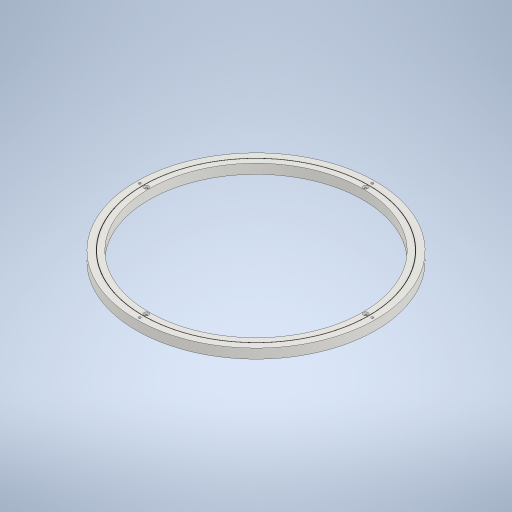
# Autodesk Inventor part: bearing_table
Saved by Autodesk Inventor 2023 (Build 270158000, 158)
## iProperties
Created: 2023-03-04
Part Number: bearing_table
Material: Generic
Document SubType Name: Modeling
Designer: caleb
Density: 1 g/cm^3
Appearance: Default
Author: caleb
Autodesk Inventor part; units mm, degrees
ref_plane "YZ Plane" through (0, 0, 0) normal (1, 0, 0) x (0, 1, 0)
ref_plane "XZ Plane" through (0, 0, 0) normal (0, 1, 0) x (-1, 0, 0)
ref_plane "XY Plane" through (0, 0, 0) normal (0, 0, 1) x (1, 0, 0)
sketch "Sketch1" plane through (0, 0, 0) normal (0, 1, 0) x (-1, 0, 0)
  circle A0 centre (0, 0) radius 111.75
  circle A1 centre (0, 0) radius 125
  circle A2 centre (0, 0) radius 117.75
  circle A3 centre (0, 0) radius 118.25
  line L0 (-111.75, 0) -> (-117.75, 0)
  line L1 (-118.25, 0) -> (-125, 0)
  point P0 (-114.75, 0)
  point P1 (-121.625, 0)
  point P2 (0, -121.625)
  point P3 (0, -114.75)
  point P4 (121.625, 0)
  point P5 (114.75, 0)
  point P6 (0, 121.625)
  point P7 (0, 114.75)
  dimension "d0" = 223.5
  dimension "d1" = 250
  dimension "d2" = 235.5
  dimension "d3" = 236.5
  dimension "d34" = 360
  constraints: 4 coincident, 4 end point, 4 horizontal alignment, 2 midpoint, 2 point on line, 1 horizontal, 17 other
extrude "Extrusion1" add sketch "Sketch1" against normal blind 10
hole "Hole3" at (114.75, 0, 0) at (0, 0, -114.75) at (0, 0, 114.75) at (-114.75, 0, 0) direction (0, -1, 0) diameter 2.4 end through all countersink diameter 5 countersink angle 90
sketch "Sketch3" plane through (0, -10, 0) normal (0, -1, 0) x (1, 0, 0)
  point P0 (0, 0)
  point P1 (0, -121.625)
  point P2 (121.625, 0)
  point P3 (0, 121.625)
  point P4 (-121.625, 0)
hole "Hole4" at (0, -10, -121.625) at (121.625, -10, 0) at (0, -10, 121.625) at (-121.625, -10, 0) direction (0, 1, 0) diameter 2.4 end through all countersink diameter 5 countersink angle 90
body "Solid1"
